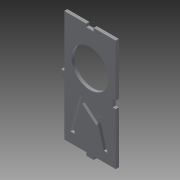
# Autodesk Inventor part: Birdhouse Tree Wall
Saved by Autodesk Inventor 2015 (Build 190159000, 159)
## iProperties
Created: 2018-03-09
Part Number: Birdhouse Tree Wall
Material: Generic
Document SubType Name: Modeling
Designer: Administrator
Density: 1 g/cm^3
Appearance: Default
Author: Administrator
Autodesk Inventor part; units mm, degrees
ref_plane "YZ Plane" through (0, 0, 0) normal (1, 0, 0) x (0, 1, 0)
ref_plane "XZ Plane" through (0, 0, 0) normal (0, 1, 0) x (-1, 0, 0)
ref_plane "XY Plane" through (0, 0, 0) normal (0, 0, 1) x (1, 0, 0)
sketch "Sketch1" plane through (0, 0, 0) normal (0, 0, 1) x (1, 0, 0)
  line L0 (0, 0) -> (52.9336, 0)
  line L1 (52.9336, 0) -> (52.9336, 114.3)
  line L2 (52.9336, 114.3) -> (0, 114.3)
  line L3 (0, 114.3) -> (0, 0)
  dimension "d0" = 114.3
  dimension "d1" = 52.9336
  constraints: 8 end point, 2 parallel, 1 horizontal, 1 perpendicular
  measures "d0" distance of L2.end L0.start
  measures "d1" distance of L0.start L0.end
extrude "Extrusion1" add sketch "Sketch1" along normal blind 3.175
sketch "Sketch2" plane through (0, 0, 3.175) normal (0, 0, 1) x (1, 0, 0)
  line L0 (0, 114.3) -> (0, 0) projected
  line L1 (52.9336, 0) -> (52.9336, 114.3) projected
  line L2 (0, 60.96) -> (-3.175, 60.96)
  line L3 (-3.175, 60.96) -> (-3.175, 53.34)
  line L4 (-3.175, 53.34) -> (0, 53.34)
  line L5 (0, 53.34) -> (0, 60.96)
  line L6 (52.9336, 60.96) -> (49.7586, 60.96)
  line L7 (49.7586, 60.96) -> (49.7586, 53.34)
  line L8 (49.7586, 53.34) -> (52.9336, 53.34)
  line L9 (52.9336, 53.34) -> (52.9336, 60.96)
  line L10 (52.9336, 114.3) -> (0, 114.3) projected
  line L11 (0, 0) -> (52.9336, 0) projected
  line L12 (30.2768, 114.3) -> (22.6568, 114.3)
  line L13 (30.2768, 0) -> (30.2768, -3.175)
  line L14 (30.2768, -3.175) -> (22.6568, -3.175)
  line L15 (22.6568, -3.175) -> (22.6568, 0)
  line L16 (22.6568, 0) -> (30.2768, 0)
  line L17 (22.6568, 114.3) -> (22.6568, 111.125)
  line L18 (22.6568, 111.125) -> (30.2768, 111.125)
  line L19 (30.2768, 111.125) -> (30.2768, 114.3)
  point P0 (0, 57.15)
  point P1 (52.9336, 57.15)
  point P2 (26.4668, 114.3)
  point P3 (26.4668, 0)
  dimension "d4" = 3.81
  dimension "d5" = 7.62
  dimension "d6" = 3.175
  dimension "d7" = 3.81
  dimension "d8" = 7.62
  dimension "d9" = 3.175
  dimension "d13" = 7.62
  dimension "d14" = 3.81
  dimension "d15" = 3.175
  dimension "d20" = 7.62
  dimension "d21" = 3.81
  dimension "d22" = 3.175
  constraints: 32 end point, 8 point on line, 7 perpendicular, 6 parallel, 4 midpoint, 2 collinear, 2 vertical
  measures "d4" distance from line of point (0, 57.15) L2
  measures "d5" distance between parallel lines of L2 L4
  measures "d6" distance between parallel lines of L0 L3
  measures "d7" distance from line of point (52.934, 57.15) L6
  measures "d8" distance between parallel lines of L6 L8
  measures "d9" distance between parallel lines of L1 L7
  measures "d13" distance between parallel lines of L13 L15
  measures "d14" distance from line of L13 point (26.467, 0)
  measures "d15" distance between parallel lines of L14 L11
  measures "d20" distance between parallel lines of L17 L19
  measures "d21" distance from line of L19 point (26.467, 114.3)
  measures "d22" distance between parallel lines of L10 L18
extrude "Extrusion2" add sketch "Sketch2" against normal blind 3.175 contours L0 L4 L3 L2 | L10 L19 L18 L17 | L11 L13 L14 L15 | L1 L8 L7 L6
extrude "Extrusion3" cut sketch "Sketch2" against normal blind 3.175 contours L10 L19 L18 L17 | L1 L8 L7 L6
sketch "Sketch3" plane through (0, 0, 3.175) normal (0, 0, 1) x (1, 0, 0)
  line L0 (0, 60.96) -> (0, 114.3)
  line L1 (22.6568, 114.3) -> (0, 114.3) projected
  line L2 (0, 114.3) -> (22.6568, 114.3)
  line L3 (22.6568, 114.3) -> (22.6568, 111.125)
  line L4 (22.6568, 111.125) -> (30.2768, 111.125)
  line L5 (30.2768, 111.125) -> (22.6568, 111.125) projected
  line L6 (30.2768, 111.125) -> (30.2768, 114.3)
  line L7 (30.2768, 114.3) -> (52.9336, 114.3)
  line L8 (52.9336, 114.3) -> (52.9336, 60.96)
  line L9 (52.9336, 60.96) -> (52.9336, 114.3) projected
  line L10 (52.9336, 60.96) -> (49.7586, 60.96)
  line L11 (49.7586, 60.96) -> (49.7586, 53.34)
  line L12 (49.7586, 60.96) -> (49.7586, 53.34) projected
  line L13 (49.7586, 53.34) -> (52.9336, 53.34)
  line L14 (52.9336, 53.34) -> (52.9336, 0)
  line L15 (52.9336, 0) -> (52.9336, 53.34) projected
  line L16 (52.9336, 0) -> (30.2768, 0)
  line L17 (0, 0) -> (22.6568, 0) projected
  line L18 (30.2768, 0) -> (30.2768, -3.175)
  line L19 (30.2768, -3.175) -> (22.6568, -3.175)
  line L20 (22.6568, -3.175) -> (30.2768, -3.175) projected
  line L21 (22.6568, -3.175) -> (22.6568, 0)
  line L22 (22.6568, 0) -> (0, 0)
  line L23 (0, 0) -> (0, 53.34)
  line L24 (0, 53.34) -> (0, 0) projected
  line L25 (0, 53.34) -> (-3.175, 53.34)
  line L26 (-3.175, 53.34) -> (-3.175, 60.96)
  line L27 (-3.175, 60.96) -> (-3.175, 53.34) projected
  line L28 (-3.175, 60.96) -> (0, 60.96)
  constraints: 40 end point, 10 perpendicular, 9 collinear
sketch "Sketch4" plane through (0, 0, 3.175) normal (0, 0, 1) x (1, 0, 0)
  circle A0 centre (26.4922, 76.2) radius 19.05
  line L0 (30.2768, 0) -> (52.9336, 0) projected
  line L1 (52.9336, 60.96) -> (52.9336, 114.3) projected
  point P0 (0, 0)
  dimension "d23" = 38.1
  dimension "d24" = 76.2
  dimension "d25" = 26.4414
  constraints: 1 centre point
  measures "d23" diameter of A0
  measures "d24" distance from line of L0 A0.centre
  measures "d25" distance from line of L1 A0.centre
sketch "Sketch5" plane through (0, 0, 3.175) normal (0, 0, 1) x (1, 0, 0)
  line L0 (6.35, 10.1986) -> (16.4034, 47.7183)
  line L1 (16.4034, 47.7183) -> (32.3606, 34.3286)
  line L2 (32.3606, 34.3286) -> (36.6232, 39.4086)
  line L3 (36.6232, 39.4086) -> (44.45, 10.1986)
  line L4 (44.45, 10.1986) -> (40.5056, 10.1986)
  line L5 (40.5056, 10.1986) -> (34.8373, 31.3529)
  line L6 (34.8373, 31.3529) -> (32.8302, 28.9609)
  line L7 (32.8302, 28.9609) -> (18.5357, 40.9555)
  line L8 (18.5357, 40.9555) -> (10.2944, 10.1986)
  line L9 (10.2944, 10.1986) -> (6.35, 10.1986)
  line L10 (0, 53.34) -> (0, 0) projected
  dimension "d26" = 3.81
  dimension "d27" = 3.81
  dimension "d29" = 3.81
  dimension "d31" = 75
  dimension "d32" = 38.1
  dimension "d33" = 6.35
  dimension "d34" = 75
  dimension "d35" = 3.81
  dimension "d36" = 29.21
  dimension "d38" = 65
  dimension "d39" = 5.08
  constraints: 20 end point, 3 parallel, 2 perpendicular, 1 collinear, 1 horizontal, 1 point on line
  measures "d26" distance between parallel lines of L0 L8
  measures "d27" distance between parallel lines of L5 L3
  measures "d29" distance between parallel lines of L1 L7
  measures "d31" angle of L9 L0
  measures "d32" distance of L3.end L0.start
  measures "d33" distance from line of L10 L0.start
  measures "d34" angle of L4 L3
  measures "d35" distance between parallel lines of L6 L2
  measures "d36" vertical distance of L2.end L3.end
  measures "d38" angle of L1 L0
  measures "d39" vertical distance of L1.end L2.end
extrude "Extrusion4" cut sketch "Sketch4" against normal blind 25.4
extrude "Extrusion5" cut sketch "Sketch5" against normal blind 2.54
body "Solid1"
